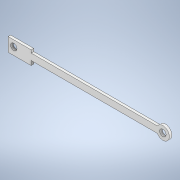
# Autodesk Inventor part: Pieza7
Saved by Autodesk Inventor 2022 (Build 260153000, 153)
## iProperties
Created: 2022-11-04
Part Number: Pieza7
Material: Resina acetálica, blanca
Document SubType Name: Modeling
Designer: Mauricio Guerrero
Density: 1.425 g/cm^3
Appearance: Suave - Blanco
Author: Mauricio Guerrero
## iProperties of the stored document Pieza7_3DPrint.ipt
Created: 2022-11-06
Part Number: Pieza7_3DPrint
Material: Genérico
Document SubType Name: Modeling
Designer: Mauricio Guerrero
Density: 1 g/cm^3
Appearance: Valor por defecto
Author: Mauricio Guerrero
Autodesk Inventor part; units mm, degrees
ref_plane "YZ Plane" through (0, 0, 0) normal (1, 0, 0) x (0, 1, 0)
ref_plane "XZ Plane" through (0, 0, 0) normal (0, 1, 0) x (-1, 0, 0)
ref_plane "XY Plane" through (0, 0, 0) normal (0, 0, 1) x (1, 0, 0)
sketch "Boceto1" plane through (0, 0, 0) normal (0, 0, 1) x (1, 0, 0)
  circle A0 centre (-1259.356, 548.7064) radius 1.25
  circle A1 centre (-1201.356, 548.7064) radius 1.25
  arc A2 (-1203.5423, 547.494) -> (-1203.4989, 549.994) centre (-1201.356, 548.7064) ccw
  line L0 (-1203.4989, 549.994) -> (-1252.6193, 549.994)
  line L1 (-1252.6193, 547.494) -> (-1203.5423, 547.494)
  line L2 (-1252.6193, 549.994) -> (-1252.6193, 551.0815)
  line L3 (-1252.6193, 551.0815) -> (-1261.5839, 551.0815)
  line L4 (-1261.5839, 551.0815) -> (-1261.5839, 545.775)
  line L5 (-1261.5839, 545.775) -> (-1252.6193, 545.775)
  line L6 (-1252.6193, 545.775) -> (-1252.6193, 547.494)
  dimension "d6" = 2.5
  dimension "d8" = 2.5
  dimension "d9" = 5
  dimension "d10" = 58
  dimension "d11" = 2.5
  constraints: 14 end point, 4 perpendicular, 3 centre point, 2 horizontal, 2 point on circle, 1 coincident, 1 point on line, 1 vertical
  measures "d6" diameter of A0
  measures "d8" diameter of A1
  measures "d9" diameter of A2
  measures "d10" distance of A1.centre A0.centre
  measures "d11" distance between parallel lines of L1 L0
extrude "Extrusión1" add sketch "Boceto1" along normal blind 1
